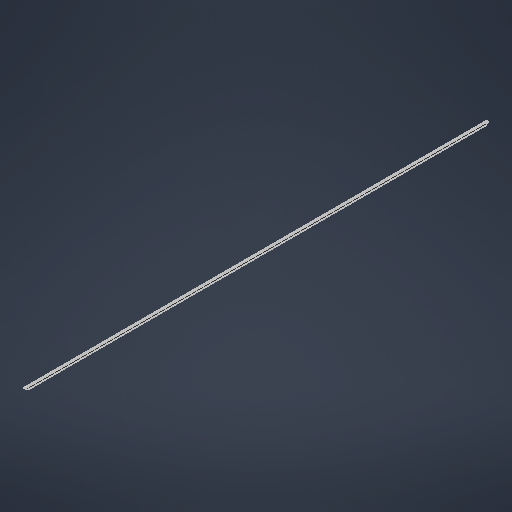
# Autodesk Inventor part: SP40-02 JUNTA EXT 2058
Saved by Autodesk Inventor 2025 (Build 290162000, 162)
## iProperties
Created: 2026-01-18
Part Number: SP40-02 JUNTA EXT 2058
Material: Caucho, negro
Document SubType Name: Modeling
Designer: ROLANDO
Density: 0.93 g/cm^3
Appearance: Caucho - Negro
Author: ROLANDO
Autodesk Inventor part; units mm, degrees
ref_plane "YZ Plane" through (0, 0, 0) normal (1, 0, 0) x (0, 1, 0)
ref_plane "XZ Plane" through (0, 0, 0) normal (0, 1, 0) x (-1, 0, 0)
sketch "Boceto1" plane through (0, 0, 0) normal (0, 0, 1) x (1, 0, 0)
  line L0 (0.6, -23) -> (0.5, -23)
  line L1 (0.5, -17.8) -> (0.6, -17.8)
  line L2 (1.1, -18.3) -> (1.1, -18.4)
  line L3 (1.6, -18.9) -> (2, -18.9)
  line L4 (1.1, -22.5) -> (1.1, -22.4)
  line L5 (1.6, -21.9) -> (2, -21.9)
  line L6 (0, -18.3) -> (0, -22.5)
  arc A0 (1.1, -18.4) -> (1.6, -18.9) centre (1.6, -18.4) ccw
  arc A1 (1.1, -18.3) -> (0.6, -17.8) centre (0.6, -18.3) ccw
  arc A2 (2, -18.9) -> (2.5, -18.4) centre (2, -18.4) ccw
  arc A3 (2.5, -22.4) -> (2, -21.9) centre (2, -22.4) ccw
  arc A4 (1.6, -21.9) -> (1.1, -22.4) centre (1.6, -22.4) ccw
  arc A5 (0.6, -23) -> (1.1, -22.5) centre (0.6, -22.5) ccw
  arc A6 (0, -22.5) -> (0.5, -23) centre (0.5, -22.5) ccw
  arc A7 (0.5, -17.8) -> (0, -18.3) centre (0.5, -18.3) ccw
  line L7 (2.5, -18.4) -> (2.5, -22.4)
  point P0 (0, -23)
  point P1 (0, -17.8)
  point P2 (1.1, -21.9)
  point P3 (0, -20.4)
  dimension "d112" = 5.2
  dimension "d115" = 2.6
  dimension "d116" = 2.6
  dimension "d117" = 1.5
  dimension "d118" = 1.5
  dimension "d119" = 3
  dimension "d125" = 1.1
  dimension "d132" = 0.5
  dimension "d133" = 0.5
  dimension "d141" = 0.5
  constraints: 16 end point, 16 point on circle, 15 tangent, 8 centre point, 7 point on line, 6 equal radius, 1 horizontal, 1 midpoint, 1 vertical
  measures "d112" distance between parallel lines of L0 L1
  measures "d115" distance from line of point (0, -20.4) L1
  measures "d116" distance from line of point (0, -20.4) L0
  measures "d117" distance from line of point (0, -20.4) L3
  measures "d118" distance from line of point (0, -20.4) L5
  measures "d119" distance between parallel lines of L5 L3
  measures "d125" distance between parallel lines of L4 L6
  measures "d132" radius of A0
  measures "d133" radius of A2
  measures "d141" radius of A6
extrude "Extrusión1" add sketch "Boceto1" against normal blind 758.2
ref_plane "Plano de trabajo2" through (0, 0, -379.1) normal (0, 0, 1) x (1, 0, 0)
sketch "Boceto2" plane through (0, -22.9, 1299.8) normal (-1, 0, 0) x (0, 0, 1)
  line L0 (-1299.8, -0.1) -> (-1299.8, 5.1)
  line L1 (-1299.8, -0.1) -> (-2058, -0.1) projected
  line L2 (-1299.8, -0.1) -> (-1305, -0.1)
  line L3 (-1299.8, 5.1) -> (-1305, -0.1)
  dimension "d146" = 45
  constraints: 6 end point, 1 coincident, 1 perpendicular, 1 point on line
  measures "d146" angle of L1 L3
extrude "Extrusión2" cut sketch "Boceto2" against normal up to surface (2.5 mm away)
mirror "Simetría1" about plane through (0, 0, -379.1) normal (0, 0, 1) of "Extrusión2"
